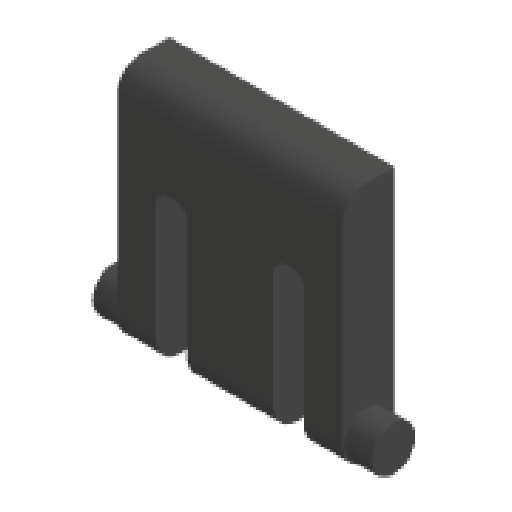
# Autodesk Inventor part: tilt_leg
Saved by Autodesk Inventor 2025 (Build 290162000, 162)
## iProperties
Created: 2025-01-10
Part Number: tilt_leg
Material: Generic
Document SubType Name: Modeling
Designer: Jan Mareš
Density: 1 g/cm^3
Appearance: Default
Author: Jan Mareš
Autodesk Inventor part; units mm, degrees
ref_plane "YZ Plane" through (0, 0, 0) normal (1, 0, 0) x (0, 1, 0)
ref_plane "XZ Plane" through (0, 0, 0) normal (0, 1, 0) x (-1, 0, 0)
ref_plane "XY Plane" through (0, 0, 0) normal (0, 0, 1) x (1, 0, 0)
sketch "Sketch1" plane through (0, 0, 0) normal (0, 0, 1) x (1, 0, 0)
  line L0 (0, -8.75) -> (0, 8.75) construction
  line L1 (-8.19, 0) -> (8.19, 0) construction
  line L2 (-5.85, -6.25) -> (5.85, -6.25)
  line L3 (5.85, -6.25) -> (5.85, 6.25)
  line L4 (5.85, 6.25) -> (-5.85, 6.25)
  line L5 (-5.85, 6.25) -> (-5.85, -6.25)
  line L6 (0, -6.25) -> (0, 6.25) construction
  point P0 (0, 0)
  dimension "d0" = 12.5
  dimension "d1" = 11.7
  constraints: 10 end point, 3 midpoint, 2 parallel, 1 horizontal, 1 perpendicular
  measures "d0" distance of L2.end L3.end
  measures "d1" distance of L3.end L4.end
extrude "Extrusion1" add sketch "Sketch1" along normal blind 2.7
sketch "Sketch3" plane through (-5.85, -6.25, 0) normal (-1, 0, 0) x (0, 0, 1)
  line L0 (0, 12.5) -> (0, 0) construction
  line L1 (0, 0) -> (2.7, 0) construction
  circle A0 centre (1.45, 1.25) radius 1.15
  line L2 (1.45, 1.25) -> (2.6, 1.25) construction
  line L3 (2.7, 12.5) -> (2.7, 0) construction
  line L4 (1.45, 1.25) -> (1.45, 0.1) construction
  point P0 (0, 6.25)
  dimension "d10" = 2.3
  dimension "d11" = 0.1
  dimension "d23" = 0.1
  constraints: 4 end point, 2 point on circle, 1 centre point, 1 horizontal, 1 parallel
  measures "d10" diameter of A0
  measures "d11" distance from line of L3 L2.end
  measures "d23" distance from line of L1 L4.end
extrude "Extrusion3" add sketch "Sketch3" along normal blind 1.4
sketch "Sketch4" plane through (0, 0, 2.7) normal (0, 0, 1) x (1, 0, 0)
  line L0 (-5.85, -6.25) -> (5.85, -6.25) construction
  line L1 (-5.85, 6.25) -> (-5.85, -6.25) construction
  line L2 (-2.25, -6.25) -> (-3.85, -6.25)
  line L3 (-3.85, -6.25) -> (-3.85, 1.75)
  line L4 (-3.85, 1.75) -> (-2.25, 1.75)
  line L5 (-2.25, 1.75) -> (-2.25, -6.25)
  point P0 (0, 0)
  dimension "d18" = 2
  dimension "d19" = 1.6
  dimension "d20" = 8
  constraints: 8 end point, 2 parallel, 1 horizontal, 1 perpendicular, 1 point on line
  measures "d18" distance between parallel lines of L1 L3
  measures "d19" distance between parallel lines of L3 L5
  measures "d20" distance of L4.end L2.start
extrude "Extrusion4" cut sketch "Sketch4" against normal through all
mirror "Mirror1" about plane through (0, 0, 0) normal (1, 0, 0) of "Extrusion3", "Extrusion4"
sketch "Sketch6" plane through (-5.85, -6.25, 0) normal (-1, 0, 0) x (0, 0, 1)
  circle A0 centre (1.45, 1.25) radius 1.15 construction
  line L0 (0, 0) -> (2.7, 0) construction
  line L1 (2.7, 12.5) -> (2.7, 0) construction
  line L2 (0, 12.5) -> (0, 0) construction
  arc A1 (1.45, 0) -> (2.7, 1.25) centre (1.45, 1.25) ccw
  line L3 (1.45, 1.25) -> (2.7, 1.25) construction
  line L4 (1.45, 1.25) -> (1.45, 0) construction
  line L5 (0, 1.25) -> (-2, 1.25)
  line L6 (-2, 1.25) -> (-2, -1.75)
  line L7 (-2, -1.75) -> (3, -1.75)
  line L8 (3, -1.75) -> (3, 1.25)
  line L9 (3, 1.25) -> (2.7, 1.25)
  arc A2 (0, 1.25) -> (1.25, 0) centre (1.25, 1.25) ccw
  line L10 (1.25, 0) -> (1.45, 0)
  line L11 (0.0201, 1.25) -> (1.25, 1.25) construction
  point P0 (0, 6.25)
  point P1 (3, 1.25)
  dimension "d32" = 3
  dimension "d34" = 3
  dimension "d49" = 0.2
  dimension "d50" = 2
  dimension "d51" = 5
  constraints: 18 end point, 4 point on circle, 4 point on line, 3 tangent, 2 centre point, 2 horizontal, 2 perpendicular, 1 collinear, 1 vertical
  measures "d32" distance of L5.end L6.end
  measures "d34" distance of L7.end L8.end
  measures "d49" distance of L4.end L10.start
  measures "d50" distance of L5.start L5.end
  measures "d51" distance of L6.end L7.end
extrude "Extrusion5" cut sketch "Sketch6" against normal through all
fillet "Fillet1" radius 0.6 4 edges at (-3.85, 1.75, 1.35) (-2.25, 1.75, 1.35) (3.85, 1.75, 1.35) (2.25, 1.75, 1.35)
fillet "Fillet3" radius 1.2 1 edges at (0, 6.25, 2.7)
body "Solid1"
